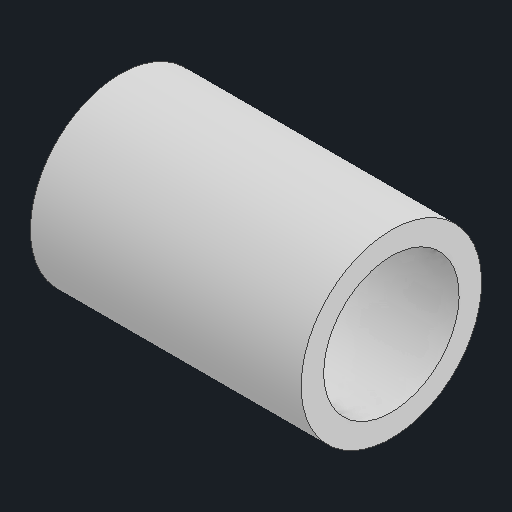
# Autodesk Inventor part: 5mm Bushing_CPY
Saved by Autodesk Inventor 2023 (Build 270158000, 158)
## iProperties
Created: 2023-02-24
Part Number: 5mm Bushing_CPY
Material: Generic
Document SubType Name: Modeling
Designer: roota
Density: 1 g/cm^3
Appearance: Default
Author: roota
Autodesk Inventor part; units mm, degrees
ref_plane "YZ Plane" through (0, 0, 0) normal (1, 0, 0) x (0, 1, 0)
ref_plane "XZ Plane" through (0, 0, 0) normal (0, 1, 0) x (-1, 0, 0)
ref_plane "XY Plane" through (0, 0, 0) normal (0, 0, 1) x (1, 0, 0)
sketch "Sketch1" plane through (0, 0, 0) normal (1, 0, 0) x (0, 1, 0)
  circle A0 centre (0, 0) radius 2
  circle A1 centre (0, 0) radius 1.5
  dimension "d0" = 4
  dimension "d1" = 3
  constraints: 2 centre point, 2 coincident
  measures "d0" diameter of A0
  measures "d1" diameter of A1
extrude "Extrusion1" add sketch "Sketch1" along normal blind 6
body "Solid1"
